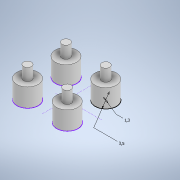
# Autodesk Inventor part: Part1
Saved by Autodesk Inventor 2021 (Build 250183000, 183)
## iProperties
Created: 2024-12-13
Part Number: Part1
Material: Generic
Document SubType Name: Modeling
Designer: 24oscnor
Density: 1 g/cm^3
Appearance: Default
Author: 24oscnor
Autodesk Inventor part; units mm, degrees
ref_plane "YZ Plane" through (0, 0, 0) normal (1, 0, 0) x (0, 1, 0)
ref_plane "XZ Plane" through (0, 0, 0) normal (0, 1, 0) x (-1, 0, 0)
ref_plane "XY Plane" through (0, 0, 0) normal (0, 0, 1) x (1, 0, 0)
sketch "Sketch1" plane through (0, 0, 0) normal (0, 1, 0) x (-1, 0, 0)
  circle A0 centre (0, 0) radius 1.75
  line L0 (-2.5887, 3.164) -> (5.0816, 3.164) construction
  circle A1 centre (0, 0) radius 0.65
  circle A2 centre (0, 6.328) radius 1.75
  circle A3 centre (0, 6.328) radius 0.65
  line L1 (3.2644, 7.3505) -> (3.2644, -3.3711) construction
  circle A4 centre (6.5289, 0) radius 1.75
  circle A5 centre (6.5289, 0) radius 0.65
  circle A6 centre (6.5289, 6.328) radius 1.75
  circle A7 centre (6.5289, 6.328) radius 0.65
  dimension "d0" = 3.5
  dimension "d1" = 1.3
  constraints: 9 symmetric about line, 8 centre point, 8 coincident, 4 end point, 1 horizontal, 1 vertical, 6 other
  measures "d0" diameter of A0
  measures "d1" diameter of A1
extrude "Extrusion1" add sketch "Sketch1" along normal blind 3
extrude "Extrusion2" add sketch "Sketch1" along normal blind 5 contours A1 | A3 | A5 | A7
body "Solid1"
